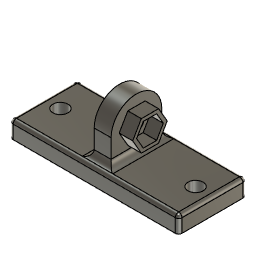
Camera Stand Part 4 (Autodesk Fusion 360 design; units mm, degrees)
Autodesk Fusion 360 part; units mm, degrees
sketch "Sketch1" plane through (0, 0, 0) normal (0, 0, 1) x (1, 0, 0)
sketch "Sketch2" plane through (0, 0, 0) normal (0, 0, 1) x (1, 0, 0)
  line L0 (-7.5, 20) -> (7.5, 20)
  line L1 (7.5, 20) -> (7.5, -20)
  line L2 (7.5, -20) -> (-7.5, -20)
  line L3 (-7.5, -20) -> (-7.5, 20)
  line L4 (-7.5, 20) -> (7.5, -20) construction
  line L5 (7.5, 20) -> (-7.5, -20) construction
  line L6 (-7.5, 2.5) -> (7.5, 2.5)
  line L7 (7.5, 2.5) -> (7.5, -2.5)
  line L8 (7.5, -2.5) -> (-7.5, -2.5)
  line L9 (-7.5, -2.5) -> (-7.5, 2.5)
  line L10 (-7.5, 2.5) -> (7.5, -2.5) construction
  line L11 (7.5, 2.5) -> (-7.5, -2.5) construction
  dimension "d1" = 15
  dimension "d2" = 40
  dimension "d3" = 5
  constraint horizontal L0
  constraint perpendicular L0 L1
  constraint parallel L0 L2
  constraint parallel L1 L3
  constraint coincident L4 origin
  constraint coincident L5 origin
  constraint horizontal L6
  constraint perpendicular L6 L7
  constraint parallel L6 L8
  constraint parallel L7 L9
  constraint coincident L10 origin
  constraint coincident L11 origin
  measures "d1" distance of L1.end L2.end
  measures "d2" distance of L0.end L1.end
  measures "d3" distance of L6.end L7.end
sketch "Sketch7" plane through (0, 0, 0) normal (0, 0, 1) x (1, 0, 0)
  line L0 (-25, 10) -> (25, 10)
  line L1 (25, 10) -> (25, -10)
  line L2 (25, -10) -> (-25, -10)
  line L3 (-25, -10) -> (-25, 10)
  line L4 (-25, 10) -> (25, -10) construction
  line L5 (25, 10) -> (-25, -10) construction
  dimension "d65" = 50
  dimension "d66" = 20
  constraint horizontal L0
  constraint perpendicular L0 L1
  constraint parallel L0 L2
  constraint parallel L1 L3
  constraint coincident L4 origin
  constraint coincident L5 origin
  measures "d65" distance of L1.end L2.end
  measures "d66" distance of L0.end L1.end
extrude "Extrude7" add sketch "Sketch7" along normal blind 5
sketch "Sketch8" plane through (0, 0, 5) normal (0, 0, 1) x (-1, 0, 0)
  line L0 (25, 10) -> (-25, 10)
  line L1 (-25, 10) -> (-25, -10)
  line L2 (-25, -10) -> (25, -10)
  line L3 (25, -10) -> (25, 10)
  line L4 (0, 0) -> (20, 0)
  dimension "d69" = 20
  constraint coincident L4.start origin
  constraint parallel L2 L4
  measures "d69" distance of L4.start L4.end
hole "Hole11" at (-20, 0, 5) direction (0, 0, -1) diameter 4.5 depth 5 tip angle 118
sketch "Sketch9" plane through (0, 0, 5) normal (0, 0, 1) x (-1, 0, 0)
  circle A0 centre (20, 0) radius 2.25
  line L0 (25, 10) -> (-25, 10)
  line L1 (-25, 10) -> (-25, -10)
  line L2 (-25, -10) -> (25, -10)
  line L3 (25, -10) -> (25, 10)
  line L4 (0, 0) -> (-20, 0)
  dimension "d73" = 20
  constraint coincident L4.start origin
  constraint horizontal L4
  measures "d73" distance of L4.start L4.end
hole "Hole12" at (20, 0, 5) direction (0, 0, -1) diameter 4.5 depth 5 tip angle 118
sketch "Sketch10" plane through (0, 0, 0) normal (0, 0, 1) x (1, 0, 0)
sketch "Sketch11" plane through (0, 0, 5) normal (0, 0, 1) x (-1, 0, 0)
  circle A0 centre (-20, 0) radius 2.25
  circle A1 centre (20, 0) radius 2.25
  line L0 (25, 10) -> (-25, 10)
  line L1 (-25, 10) -> (-25, -10)
  line L2 (-25, -10) -> (25, -10)
  line L3 (25, -10) -> (25, 10)
  line L4 (2.5, 7.5) -> (-2.5, 7.5)
  line L5 (-2.5, 7.5) -> (-2.5, -7.5)
  line L6 (-2.5, -7.5) -> (2.5, -7.5)
  line L7 (2.5, -7.5) -> (2.5, 7.5)
  line L8 (2.5, 7.5) -> (-2.5, -7.5) construction
  line L9 (-2.5, 7.5) -> (2.5, -7.5) construction
  dimension "d77" = 5
  dimension "d78" = 15
  constraint horizontal L4
  constraint perpendicular L4 L5
  constraint parallel L4 L6
  constraint parallel L5 L7
  constraint coincident L8 origin
  constraint coincident L9 origin
  measures "d77" distance of L5.end L6.end
  measures "d78" distance of L4.end L5.end
extrude "Extrude8" add sketch "Sketch11" along normal blind 15 contours L4 L5 L6 L7
fillet "Fillet4" radius 7.5 2 edges at (0, -7.5, 20) (0, 7.5, 20)
hole "Hole13" at (2.5, 0, 12.5) direction (-1, 0, 0) diameter 4.5 depth 5 tip angle 118
fillet "Fillet5" radius 1 4 edges at (-25, 0, 5) (0, 10, 5) (0, -10, 5) (25, 0, 5)
fillet "Fillet6" radius 1 8 edges at (25, -10, 2) (24.7071, -9.7071, 4.7071) (-25, -10, 2) (-24.7071, -9.7071, 4.7071) (-25, 10, 2) (-24.7071, 9.7071, 4.7071) (25, 10, 2) (24.7071, 9.7071, 4.7071)
fillet "Fillet7" radius 2 4 edges at (0, -7.5, 5) (2.5, 0, 5) (0, 7.5, 5) (-2.5, 0, 5)
sketch "Sketch12" plane through (2.5, 0, 0) normal (1, 0, 0) x (0, 1, 0)
  line L0 (-7.5, 7) -> (7.5, 7)
  line L1 (7.5, 7) -> (7.5, 12.5)
  arc A0 (7.5, 12.5) -> (-7.5, 12.5) centre (0, 12.5) ccw
  line L2 (-7.5, 12.5) -> (-7.5, 7)
  circle A1 centre (0, 12.5) radius 2.25
  line L3 (3.9548, 12.5) -> (1.9774, 15.925)
  line L4 (1.9774, 15.925) -> (-1.9774, 15.925)
  line L5 (-1.9774, 15.925) -> (-3.9548, 12.5)
  line L6 (-3.9548, 12.5) -> (-1.9774, 9.075)
  line L7 (-1.9774, 9.075) -> (1.9774, 9.075)
  line L8 (1.9774, 9.075) -> (3.9548, 12.5)
  line L9 (-5.1095, 12.5) -> (-2.5548, 8.075)
  line L10 (-2.5548, 8.075) -> (2.5548, 8.075)
  line L11 (2.5548, 8.075) -> (5.1095, 12.5)
  line L12 (5.1095, 12.5) -> (2.5548, 16.925)
  line L13 (2.5548, 16.925) -> (-2.5548, 16.925)
  line L14 (-2.5548, 16.925) -> (-5.1095, 12.5)
  point P0 (0, 12.5)
  dimension "d92" = 6.85
  dimension "d93" = 1
  constraint coincident P0 A0.centre
  constraint horizontal L4
  measures "d92" distance of L4 L7
extrude "Extrude9" add sketch "Sketch12" along normal blind 4 contours L9 L10 L11 L12 L13 L14
sketch "Sketch3" plane through (0, 0, 0) normal (0, 0, 1) x (1, 0, 0)
  line L0 (-7.5, 2.5) -> (7.5, 2.5)
  line L1 (7.5, 2.5) -> (7.5, -2.5)
  line L2 (7.5, -2.5) -> (-7.5, -2.5)
  line L3 (-7.5, -2.5) -> (-7.5, 2.5)
  line L4 (-7.5, 2.5) -> (7.5, -2.5) construction
  line L5 (7.5, 2.5) -> (-7.5, -2.5) construction
  dimension "d6" = 15
  dimension "d7" = 5
  constraint horizontal L0
  constraint perpendicular L0 L1
  constraint parallel L0 L2
  constraint parallel L1 L3
  constraint coincident L4 origin
  constraint coincident L5 origin
  measures "d6" distance of L1.end L2.end
  measures "d7" distance of L0.end L1.end
extrude "Extrude2" [suppressed]
hole "Hole1" [suppressed]
sketch "Sketch4" plane through (0, 0, 0) normal (0, 0, 1) x (1, 0, 0)
ref_plane "WorkPlane1" through (0, 0, 5) normal (0, 0, 1) x (1, 0, 0)
sketch "Sketch5" plane through (0, 0, 5) normal (0, 0, 1) x (1, 0, 0)
  line L0 (0, 0) -> (0, 10)
  line L1 (-7.5, 12.5) -> (7.5, 12.5)
  line L2 (7.5, 12.5) -> (7.5, 7.5)
  line L3 (7.5, 7.5) -> (-7.5, 7.5)
  line L4 (-7.5, 7.5) -> (-7.5, 12.5)
  line L5 (-7.5, 12.5) -> (7.5, 7.5) construction
  line L6 (7.5, 12.5) -> (-7.5, 7.5) construction
  point P0 (0, 10)
  dimension "d17" = 10
  dimension "d18" = 15
  dimension "d19" = 5
  constraint coincident L0.start origin
  constraint vertical L0
  constraint horizontal L1
  constraint perpendicular L1 L2
  constraint parallel L1 L3
  constraint parallel L2 L4
  constraint coincident L5 P0
  constraint coincident L6 P0
  constraint coincident P0 L0.end
  measures "d17" distance of L0.start P0
  measures "d18" distance of L2.end L3.end
  measures "d19" distance of L1.end L2.end
hole "Hole2" [suppressed]
ref_plane "WorkPlane2" through (0, 0, 5) normal (0, 0, 1) x (1, 0, 0)
sketch "Sketch6" plane through (0, 0, 5) normal (0, 0, 1) x (1, 0, 0)
  line L0 (0, 0) -> (0, -10)
  line L1 (7.5, -12.5) -> (-7.5, -12.5)
  line L2 (-7.5, -12.5) -> (-7.5, -7.5)
  line L3 (-7.5, -7.5) -> (7.5, -7.5)
  line L4 (7.5, -7.5) -> (7.5, -12.5)
  line L5 (7.5, -12.5) -> (-7.5, -7.5) construction
  line L6 (-7.5, -12.5) -> (7.5, -7.5) construction
  point P0 (0, -10)
  dimension "d30" = 10
  dimension "d31" = 15
  dimension "d32" = 5
  constraint coincident L0.start origin
  constraint vertical L0
  constraint horizontal L1
  constraint perpendicular L1 L2
  constraint parallel L1 L3
  constraint parallel L2 L4
  constraint coincident L5 P0
  constraint coincident L6 P0
  constraint coincident P0 L0.end
  measures "d30" distance of L0.start P0
  measures "d31" distance of L2.end L3.end
  measures "d32" distance of L1.end L2.end
hole "Hole3" [suppressed]
delete_face "DeleteFace1" [suppressed]
delete_face "DeleteFace2" [suppressed]
delete_face "DeleteFace3" [suppressed]
hole "Hole6" [suppressed]
hole "Hole7" [suppressed]
hole "Hole8" [suppressed]
extrude "Extrude5" [suppressed]
extrude "Extrude6" [suppressed]
